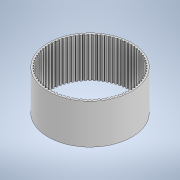
# Autodesk Inventor part: Closed Loop GT-2 (parametric)
Saved by Autodesk Inventor 2020.3 (Build 243373000, 373)
## iProperties
Created: 2021-02-16
Part Number: Closed Loop GT-2 (parametric)
Material: Generic
Document SubType Name: Modeling
Designer: juanp
Density: 1 g/cm^3
Appearance: Default
Author: juanp
Autodesk Inventor part; units mm, degrees
(part 1 of 2)
ref_plane "YZ Plane" through (0, 0, 0) normal (1, 0, 0) x (0, 1, 0)
ref_plane "XZ Plane" through (0, 0, 0) normal (0, 1, 0) x (-1, 0, 0)
ref_plane "XY Plane" through (0, 0, 0) normal (0, 0, 1) x (1, 0, 0)
sketch "Sketch1" plane through (0, 0, 0) normal (0, 1, 0) x (-1, 0, 0)
  circle A0 centre (0, 0) radius 26.3648
  circle A1 centre (0, 0) radius 25.4648
  line L0 (25.4648, 0) -> (24.7148, 0) construction
  arc A2 (25.0266, 0.4989) -> (24.7148, 0) centre (25.2698, 0) ccw
  arc A3 (25.325, 0.5902) -> (25.0266, 0.4989) centre (25.4648, -0.4) ccw
  arc A4 (25.325, 0.5902) -> (25.4539, 0.7431) centre (25.304, 0.7387) ccw
  line L1 (24.7148, 0) -> (0, 0)
  arc A5 (24.7148, 0) -> (25.0266, -0.4989) centre (25.2698, 0) ccw
  arc A6 (25.0266, -0.4989) -> (25.325, -0.5902) centre (25.4648, 0.4) ccw
  arc A7 (25.4539, -0.7431) -> (25.325, -0.5902) centre (25.304, -0.7387) ccw
  arc A8 (25.4338, 1.2563) -> (25.2932, 1.3986) centre (25.284, 1.2489) ccw
  arc A9 (24.9886, 1.4662) -> (25.2932, 1.3986) centre (25.3549, 2.3967) ccw
  arc A10 (24.6386, 1.9391) -> (24.9886, 1.4662) centre (25.1919, 1.9826) ccw
  line L2 (25.3863, 1.9979) -> (24.6386, 1.9391) construction
  arc A11 (25.2006, 2.5753) -> (24.9103, 2.4609) centre (25.4177, 1.5992) ccw
  arc A12 (24.9103, 2.4609) -> (24.6386, 1.9391) centre (25.1919, 1.9826) ccw
  arc A13 (25.2006, 2.5753) -> (25.3172, 2.7379) centre (25.168, 2.7218) ccw
  arc A14 (25.2568, 3.2479) -> (25.1055, 3.3788) centre (25.108, 3.2288) ccw
  arc A15 (24.7965, 3.4223) -> (25.1055, 3.3788) centre (25.0887, 4.3786) ccw
  arc A16 (24.4105, 3.8662) -> (24.7965, 3.4223) centre (24.9587, 3.9531) ccw
  line L3 (25.1513, 3.9836) -> (24.4105, 3.8662) construction
  arc A17 (24.9209, 4.5446) -> (24.6404, 4.4078) centre (25.2139, 3.5885) ccw
  arc A18 (24.6404, 4.4078) -> (24.4105, 3.8662) centre (24.9587, 3.9531) ccw
  arc A19 (24.9209, 4.5446) -> (25.0243, 4.7158) centre (24.8769, 4.688) ccw
  arc A20 (24.9241, 5.2196) -> (24.763, 5.3381) centre (24.7773, 5.1888) ccw
  arc A21 (24.4516, 5.3572) -> (24.763, 5.3381) centre (24.6678, 6.3336) ccw
  arc A22 (24.0319, 5.7696) -> (24.4516, 5.3572) centre (24.5716, 5.8991) ccw
  line L4 (24.7612, 5.9446) -> (24.0319, 5.7696) construction
  arc A23 (24.4875, 6.4859) -> (24.2186, 6.3274) centre (24.8546, 5.5557) ccw
  arc A24 (24.2186, 6.3274) -> (24.0319, 5.7696) centre (24.5716, 5.8991) ccw
  arc A25 (24.4875, 6.4859) -> (24.5772, 6.6647) centre (24.4324, 6.6254) ccw
  arc A26 (24.4378, 7.159) -> (24.2679, 7.2646) centre (24.2938, 7.1168) ccw
  arc A27 (23.9559, 7.2592) -> (24.2679, 7.2646) centre (24.0948, 8.2495) ccw
  arc A28 (23.5052, 7.6373) -> (23.9559, 7.2592) centre (24.033, 7.8088) ccw
  line L5 (24.2185, 7.8691) -> (23.5052, 7.6373) construction
  arc A29 (23.9031, 8.3871) -> (23.6475, 8.2081) centre (24.3421, 7.4886) ccw
  arc A30 (23.6475, 8.2081) -> (23.5052, 7.6373) centre (24.033, 7.8088) ccw
  arc A31 (23.9031, 8.3871) -> (23.9785, 8.5724) centre (23.8373, 8.5219) ccw
  arc A32 (23.8007, 9.0543) -> (23.6231, 9.1462) centre (23.6605, 9.001) ccw
  arc A33 (23.3125, 9.1164) -> (23.6231, 9.1462) centre (23.3733, 10.1145) ccw
  arc A34 (22.8335, 9.4579) -> (23.3125, 9.1164) centre (23.3462, 9.6703) ccw
  line L6 (23.5264, 9.745) -> (22.8335, 9.4579) construction
  arc A35 (23.1714, 10.2367) -> (22.9306, 10.0382) centre (23.6795, 9.3754) ccw
  arc A36 (22.9306, 10.0382) -> (22.8335, 9.4579) centre (23.3462, 9.6703) ccw
  arc A37 (23.1714, 10.2367) -> (23.232, 10.4273) centre (23.0952, 10.3659) ccw
  arc A38 (23.017, 10.8938) -> (22.8327, 10.9714) centre (22.8814, 10.8296) ccw
  arc A39 (22.5253, 10.9173) -> (22.8327, 10.9714) centre (22.5077, 11.9172) ccw
  arc A40 (22.021, 11.2203) -> (22.5253, 10.9173) centre (22.5155, 11.4722) ccw
  line L7 (22.6893, 11.5608) -> (22.021, 11.2203) construction
  arc A41 (22.2968, 12.0232) -> (22.0724, 11.8063) centre (22.8709, 11.2044) ccw
  arc A42 (22.0724, 11.8063) -> (22.021, 11.2203) centre (22.5155, 11.4722) ccw
  arc A43 (22.2968, 12.0232) -> (22.3423, 12.2179) centre (22.2107, 12.146) ccw
  arc A44 (22.0913, 12.6661) -> (21.9015, 12.7291) centre (21.9612, 12.5915) ccw
  arc A45 (21.5993, 12.651) -> (21.9015, 12.7291) centre (21.5033, 13.6464) ccw
  arc A46 (21.0728, 12.9134) -> (21.5993, 12.651) centre (21.546, 13.2034) ccw
  line L8 (21.7123, 13.3053) -> (21.0728, 12.9134) construction
  arc A47 (21.2847, 13.7355) -> (21.078, 13.5017) centre (21.9213, 12.9643) ccw
  arc A48 (21.078, 13.5017) -> (21.0728, 12.9134) centre (21.546, 13.2034) ccw
  arc A49 (21.2847, 13.7355) -> (21.3148, 13.9332) centre (21.1892, 13.8512) ccw
  arc A50 (21.0294, 14.3603) -> (20.8352, 14.4082) centre (20.9056, 14.2757) ccw
  arc A51 (20.5402, 14.3067) -> (20.8352, 14.4082) centre (20.3663, 15.2914) ccw
  arc A52 (19.9947, 14.527) -> (20.5402, 14.3067) centre (20.4437, 14.8532) ccw
  line L9 (20.6014, 14.9678) -> (19.9947, 14.527) construction
  arc A53 (20.1414, 15.3631) -> (19.9537, 15.1139) centre (20.8366, 14.6442) ccw
  arc A54 (19.9537, 15.1139) -> (19.9947, 14.527) centre (20.4437, 14.8532) ccw
  arc A55 (20.1414, 15.3631) -> (20.1559, 15.5626) centre (20.0372, 15.4709) ccw
  arc A56 (19.8379, 15.966) -> (19.6406, 15.9985) centre (19.7211, 15.8719) ccw
  arc A57 (19.3544, 15.8741) -> (19.6406, 15.9985) centre (19.1038, 16.8422) ccw
  arc A58 (18.7933, 16.051) -> (19.3544, 15.8741) centre (19.2153, 16.4114) ccw
  line L10 (19.3636, 16.5381) -> (18.7933, 16.051) construction
  arc A59 (18.874, 16.896) -> (18.7064, 16.6328) centre (19.6234, 16.2339) ccw
  arc A60 (18.7064, 16.6328) -> (18.7933, 16.051) centre (19.2153, 16.4114) ccw
  arc A61 (18.874, 16.896) -> (18.8727, 17.0961) centre (18.7616, 16.9954) ccw
  arc A62 (18.5241, 17.4732) -> (18.3248, 17.4901) centre (18.415, 17.3703) ccw
  arc A63 (18.0492, 17.3437) -> (18.3248, 17.4901) centre (17.7235, 18.2892) ccw
  arc A64 (17.476, 17.476) -> (18.0492, 17.3437) centre (17.8684, 17.8684) ccw
  line L11 (18.0063, 18.0063) -> (17.476, 17.476) construction
  arc A65 (17.4901, 18.3248) -> (17.3437, 18.0492) centre (18.2892, 17.7235) ccw
  arc A66 (17.3437, 18.0492) -> (17.476, 17.476) centre (17.8684, 17.8684) ccw
  arc A67 (17.4901, 18.3248) -> (17.4732, 18.5241) centre (17.3703, 18.415) ccw
  arc A68 (17.0961, 18.8727) -> (16.896, 18.874) centre (16.9954, 18.7616) ccw
  arc A69 (16.6328, 18.7064) -> (16.896, 18.874) centre (16.2339, 19.6234) ccw
  arc A70 (16.051, 18.7933) -> (16.6328, 18.7064) centre (16.4114, 19.2153) ccw
  line L12 (16.5381, 19.3636) -> (16.051, 18.7933) construction
  arc A71 (15.9985, 19.6406) -> (15.8741, 19.3544) centre (16.8422, 19.1038) ccw
  arc A72 (15.8741, 19.3544) -> (16.051, 18.7933) centre (16.4114, 19.2153) ccw
  arc A73 (15.9985, 19.6406) -> (15.966, 19.8379) centre (15.8719, 19.7211) ccw
  arc A74 (15.5626, 20.1559) -> (15.3631, 20.1414) centre (15.4709, 20.0372) ccw
  arc A75 (15.1139, 19.9537) -> (15.3631, 20.1414) centre (14.6442, 20.8366) ccw
  arc A76 (14.527, 19.9947) -> (15.1139, 19.9537) centre (14.8532, 20.4437) ccw
  line L13 (14.9678, 20.6014) -> (14.527, 19.9947) construction
  arc A77 (14.4082, 20.8352) -> (14.3067, 20.5402) centre (15.2914, 20.3663) ccw
  arc A78 (14.3067, 20.5402) -> (14.527, 19.9947) centre (14.8532, 20.4437) ccw
  arc A79 (14.4082, 20.8352) -> (14.3603, 21.0294) centre (14.2757, 20.9056) ccw
  arc A80 (13.9332, 21.3148) -> (13.7355, 21.2847) centre (13.8512, 21.1892) ccw
  arc A81 (13.5017, 21.078) -> (13.7355, 21.2847) centre (12.9643, 21.9213) ccw
  arc A82 (12.9134, 21.0728) -> (13.5017, 21.078) centre (13.2034, 21.546) ccw
  line L14 (13.3053, 21.7123) -> (12.9134, 21.0728) construction
  arc A83 (12.7291, 21.9015) -> (12.651, 21.5993) centre (13.6464, 21.5033) ccw
  arc A84 (12.651, 21.5993) -> (12.9134, 21.0728) centre (13.2034, 21.546) ccw
  arc A85 (12.7291, 21.9015) -> (12.6661, 22.0913) centre (12.5915, 21.9612) ccw
  arc A86 (12.2179, 22.3423) -> (12.0232, 22.2968) centre (12.146, 22.2107) ccw
  arc A87 (11.8063, 22.0724) -> (12.0232, 22.2968) centre (11.2044, 22.8709) ccw
  arc A88 (11.2203, 22.021) -> (11.8063, 22.0724) centre (11.4722, 22.5155) ccw
  line L15 (11.5608, 22.6893) -> (11.2203, 22.021) construction
  arc A89 (10.9714, 22.8327) -> (10.9173, 22.5253) centre (11.9172, 22.5077) ccw
  arc A90 (10.9173, 22.5253) -> (11.2203, 22.021) centre (11.4722, 22.5155) ccw
  arc A91 (10.9714, 22.8327) -> (10.8938, 23.017) centre (10.8296, 22.8814) ccw
  arc A92 (10.4273, 23.232) -> (10.2367, 23.1714) centre (10.3659, 23.0952) ccw
  arc A93 (10.0382, 22.9306) -> (10.2367, 23.1714) centre (9.3754, 23.6795) ccw
  arc A94 (9.4579, 22.8335) -> (10.0382, 22.9306) centre (9.6703, 23.3462) ccw
  line L16 (9.745, 23.5264) -> (9.4579, 22.8335) construction
  arc A95 (9.1462, 23.6231) -> (9.1164, 23.3125) centre (10.1145, 23.3733) ccw
  arc A96 (9.1164, 23.3125) -> (9.4579, 22.8335) centre (9.6703, 23.3462) ccw
  arc A97 (9.1462, 23.6231) -> (9.0543, 23.8007) centre (9.001, 23.6605) ccw
  arc A98 (8.5724, 23.9785) -> (8.3871, 23.9031) centre (8.5219, 23.8373) ccw
  arc A99 (8.2081, 23.6475) -> (8.3871, 23.9031) centre (7.4886, 24.3421) ccw
  arc A100 (7.6373, 23.5052) -> (8.2081, 23.6475) centre (7.8088, 24.033) ccw
  line L17 (7.8691, 24.2185) -> (7.6373, 23.5052) construction
  arc A101 (7.2646, 24.2679) -> (7.2592, 23.9559) centre (8.2495, 24.0948) ccw
  arc A102 (7.2592, 23.9559) -> (7.6373, 23.5052) centre (7.8088, 24.033) ccw
  arc A103 (7.2646, 24.2679) -> (7.159, 24.4378) centre (7.1168, 24.2938) ccw
  arc A104 (6.6647, 24.5772) -> (6.4859, 24.4875) centre (6.6254, 24.4324) ccw
  arc A105 (6.3274, 24.2186) -> (6.4859, 24.4875) centre (5.5557, 24.8546) ccw
  arc A106 (5.7696, 24.0319) -> (6.3274, 24.2186) centre (5.8991, 24.5716) ccw
  line L18 (5.9446, 24.7612) -> (5.7696, 24.0319) construction
  arc A107 (5.3381, 24.763) -> (5.3572, 24.4516) centre (6.3336, 24.6678) ccw
  arc A108 (5.3572, 24.4516) -> (5.7696, 24.0319) centre (5.8991, 24.5716) ccw
  arc A109 (5.3381, 24.763) -> (5.2196, 24.9241) centre (5.1888, 24.7773) ccw
  arc A110 (4.7158, 25.0243) -> (4.5446, 24.9209) centre (4.688, 24.8769) ccw
  arc A111 (4.4078, 24.6404) -> (4.5446, 24.9209) centre (3.5885, 25.2139) ccw
  arc A112 (3.8662, 24.4105) -> (4.4078, 24.6404) centre (3.9531, 24.9587) ccw
  line L19 (3.9836, 25.1513) -> (3.8662, 24.4105) construction
  arc A113 (3.3788, 25.1055) -> (3.4223, 24.7965) centre (4.3786, 25.0887) ccw
  arc A114 (3.4223, 24.7965) -> (3.8662, 24.4105) centre (3.9531, 24.9587) ccw
  arc A115 (3.3788, 25.1055) -> (3.2479, 25.2568) centre (3.2288, 25.108) ccw
  arc A116 (2.7379, 25.3172) -> (2.5753, 25.2006) centre (2.7218, 25.168) ccw
  arc A117 (2.4609, 24.9103) -> (2.5753, 25.2006) centre (1.5992, 25.4177) ccw
  arc A118 (1.9391, 24.6386) -> (2.4609, 24.9103) centre (1.9826, 25.1919) ccw
  line L20 (1.9979, 25.3863) -> (1.9391, 24.6386) construction
  arc A119 (1.3986, 25.2932) -> (1.4662, 24.9886) centre (2.3967, 25.3549) ccw
  arc A120 (1.4662, 24.9886) -> (1.9391, 24.6386) centre (1.9826, 25.1919) ccw
  arc A121 (1.3986, 25.2932) -> (1.2563, 25.4338) centre (1.2489, 25.284) ccw
  arc A122 (0.7431, 25.4539) -> (0.5902, 25.325) centre (0.7387, 25.304) ccw
  arc A123 (0.4989, 25.0266) -> (0.5902, 25.325) centre (-0.4, 25.4648) ccw
  arc A124 (0, 24.7148) -> (0.4989, 25.0266) centre (0, 25.2698) ccw
  line L21 (0, 25.4648) -> (0, 24.7148) construction
  arc A125 (-0.5902, 25.325) -> (-0.4989, 25.0266) centre (0.4, 25.4648) ccw
  arc A126 (-0.4989, 25.0266) -> (0, 24.7148) centre (0, 25.2698) ccw
  arc A127 (-0.5902, 25.325) -> (-0.7431, 25.4539) centre (-0.7387, 25.304) ccw
  arc A128 (-1.2563, 25.4338) -> (-1.3986, 25.2932) centre (-1.2489, 25.284) ccw
  arc A129 (-1.4662, 24.9886) -> (-1.3986, 25.2932) centre (-2.3967, 25.3549) ccw
  arc A130 (-1.9391, 24.6386) -> (-1.4662, 24.9886) centre (-1.9826, 25.1919) ccw
  line L22 (-1.9979, 25.3863) -> (-1.9391, 24.6386) construction
  arc A131 (-2.5753, 25.2006) -> (-2.4609, 24.9103) centre (-1.5992, 25.4177) ccw
  arc A132 (-2.4609, 24.9103) -> (-1.9391, 24.6386) centre (-1.9826, 25.1919) ccw
  arc A133 (-2.5753, 25.2006) -> (-2.7379, 25.3172) centre (-2.7218, 25.168) ccw
  arc A134 (-3.2479, 25.2568) -> (-3.3788, 25.1055) centre (-3.2288, 25.108) ccw
  arc A135 (-3.4223, 24.7965) -> (-3.3788, 25.1055) centre (-4.3786, 25.0887) ccw
  arc A136 (-3.8662, 24.4105) -> (-3.4223, 24.7965) centre (-3.9531, 24.9587) ccw
  line L23 (-3.9836, 25.1513) -> (-3.8662, 24.4105) construction
  arc A137 (-4.5446, 24.9209) -> (-4.4078, 24.6404) centre (-3.5885, 25.2139) ccw
  arc A138 (-4.4078, 24.6404) -> (-3.8662, 24.4105) centre (-3.9531, 24.9587) ccw
  arc A139 (-4.5446, 24.9209) -> (-4.7158, 25.0243) centre (-4.688, 24.8769) ccw
  arc A140 (-5.2196, 24.9241) -> (-5.3381, 24.763) centre (-5.1888, 24.7773) ccw
  arc A141 (-5.3572, 24.4516) -> (-5.3381, 24.763) centre (-6.3336, 24.6678) ccw
  arc A142 (-5.7696, 24.0319) -> (-5.3572, 24.4516) centre (-5.8991, 24.5716) ccw
  line L24 (-5.9446, 24.7612) -> (-5.7696, 24.0319) construction
  arc A143 (-6.4859, 24.4875) -> (-6.3274, 24.2186) centre (-5.5557, 24.8546) ccw
  arc A144 (-6.3274, 24.2186) -> (-5.7696, 24.0319) centre (-5.8991, 24.5716) ccw
  arc A145 (-6.4859, 24.4875) -> (-6.6647, 24.5772) centre (-6.6254, 24.4324) ccw
  arc A146 (-7.159, 24.4378) -> (-7.2646, 24.2679) centre (-7.1168, 24.2938) ccw
  arc A147 (-7.2592, 23.9559) -> (-7.2646, 24.2679) centre (-8.2495, 24.0948) ccw
  arc A148 (-7.6373, 23.5052) -> (-7.2592, 23.9559) centre (-7.8088, 24.033) ccw
  line L25 (-7.8691, 24.2185) -> (-7.6373, 23.5052) construction
  arc A149 (-8.3871, 23.9031) -> (-8.2081, 23.6475) centre (-7.4886, 24.3421) ccw
  arc A150 (-8.2081, 23.6475) -> (-7.6373, 23.5052) centre (-7.8088, 24.033) ccw
  arc A151 (-8.3871, 23.9031) -> (-8.5724, 23.9785) centre (-8.5219, 23.8373) ccw
  arc A152 (-9.0543, 23.8007) -> (-9.1462, 23.6231) centre (-9.001, 23.6605) ccw
  arc A153 (-9.1164, 23.3125) -> (-9.1462, 23.6231) centre (-10.1145, 23.3733) ccw
  arc A154 (-9.4579, 22.8335) -> (-9.1164, 23.3125) centre (-9.6703, 23.3462) ccw
  line L26 (-9.745, 23.5264) -> (-9.4579, 22.8335) construction
  arc A155 (-10.2367, 23.1714) -> (-10.0382, 22.9306) centre (-9.3754, 23.6795) ccw
  arc A156 (-10.0382, 22.9306) -> (-9.4579, 22.8335) centre (-9.6703, 23.3462) ccw
  arc A157 (-10.2367, 23.1714) -> (-10.4273, 23.232) centre (-10.3659, 23.0952) ccw
  arc A158 (-10.8938, 23.017) -> (-10.9714, 22.8327) centre (-10.8296, 22.8814) ccw
  arc A159 (-10.9173, 22.5253) -> (-10.9714, 22.8327) centre (-11.9172, 22.5077) ccw
  arc A160 (-11.2203, 22.021) -> (-10.9173, 22.5253) centre (-11.4722, 22.5155) ccw
  line L27 (-11.5608, 22.6893) -> (-11.2203, 22.021) construction
  arc A161 (-12.0232, 22.2968) -> (-11.8063, 22.0724) centre (-11.2044, 22.8709) ccw
  arc A162 (-11.8063, 22.0724) -> (-11.2203, 22.021) centre (-11.4722, 22.5155) ccw
  arc A163 (-12.0232, 22.2968) -> (-12.2179, 22.3423) centre (-12.146, 22.2107) ccw
  arc A164 (-12.6661, 22.0913) -> (-12.7291, 21.9015) centre (-12.5915, 21.9612) ccw
  arc A165 (-12.651, 21.5993) -> (-12.7291, 21.9015) centre (-13.6464, 21.5033) ccw
  arc A166 (-12.9134, 21.0728) -> (-12.651, 21.5993) centre (-13.2034, 21.546) ccw
  line L28 (-13.3053, 21.7123) -> (-12.9134, 21.0728) construction
  arc A167 (-13.7355, 21.2847) -> (-13.5017, 21.078) centre (-12.9643, 21.9213) ccw
  arc A168 (-13.5017, 21.078) -> (-12.9134, 21.0728) centre (-13.2034, 21.546) ccw
  arc A169 (-13.7355, 21.2847) -> (-13.9332, 21.3148) centre (-13.8512, 21.1892) ccw
  arc A170 (-14.3603, 21.0294) -> (-14.4082, 20.8352) centre (-14.2757, 20.9056) ccw
  arc A171 (-14.3067, 20.5402) -> (-14.4082, 20.8352) centre (-15.2914, 20.3663) ccw
  arc A172 (-14.527, 19.9947) -> (-14.3067, 20.5402) centre (-14.8532, 20.4437) ccw
  line L29 (-14.9678, 20.6014) -> (-14.527, 19.9947) construction
  arc A173 (-15.3631, 20.1414) -> (-15.1139, 19.9537) centre (-14.6442, 20.8366) ccw
  arc A174 (-15.1139, 19.9537) -> (-14.527, 19.9947) centre (-14.8532, 20.4437) ccw
  arc A175 (-15.3631, 20.1414) -> (-15.5626, 20.1559) centre (-15.4709, 20.0372) ccw
  arc A176 (-15.966, 19.8379) -> (-15.9985, 19.6406) centre (-15.8719, 19.7211) ccw
  arc A177 (-15.8741, 19.3544) -> (-15.9985, 19.6406) centre (-16.8422, 19.1038) ccw
  arc A178 (-16.051, 18.7933) -> (-15.8741, 19.3544) centre (-16.4114, 19.2153) ccw
  line L30 (-16.5381, 19.3636) -> (-16.051, 18.7933) construction
  arc A179 (-16.896, 18.874) -> (-16.6328, 18.7064) centre (-16.2339, 19.6234) ccw
  arc A180 (-16.6328, 18.7064) -> (-16.051, 18.7933) centre (-16.4114, 19.2153) ccw
  arc A181 (-16.896, 18.874) -> (-17.0961, 18.8727) centre (-16.9954, 18.7616) ccw
  arc A182 (-17.4732, 18.5241) -> (-17.4901, 18.3248) centre (-17.3703, 18.415) ccw
  arc A183 (-17.3437, 18.0492) -> (-17.4901, 18.3248) centre (-18.2892, 17.7235) ccw
  arc A184 (-17.476, 17.476) -> (-17.3437, 18.0492) centre (-17.8684, 17.8684) ccw
  line L31 (-18.0063, 18.0063) -> (-17.476, 17.476) construction
  arc A185 (-18.3248, 17.4901) -> (-18.0492, 17.3437) centre (-17.7235, 18.2892) ccw
  arc A186 (-18.0492, 17.3437) -> (-17.476, 17.476) centre (-17.8684, 17.8684) ccw
  arc A187 (-18.3248, 17.4901) -> (-18.5241, 17.4732) centre (-18.415, 17.3703) ccw
  arc A188 (-18.8727, 17.0961) -> (-18.874, 16.896) centre (-18.7616, 16.9954) ccw
  arc A189 (-18.7064, 16.6328) -> (-18.874, 16.896) centre (-19.6234, 16.2339) ccw
  arc A190 (-18.7933, 16.051) -> (-18.7064, 16.6328) centre (-19.2153, 16.4114) ccw
  line L32 (-19.3636, 16.5381) -> (-18.7933, 16.051) construction
  arc A191 (-19.6406, 15.9985) -> (-19.3544, 15.8741) centre (-19.1038, 16.8422) ccw
  arc A192 (-19.3544, 15.8741) -> (-18.7933, 16.051) centre (-19.2153, 16.4114) ccw
  arc A193 (-19.6406, 15.9985) -> (-19.8379, 15.966) centre (-19.7211, 15.8719) ccw
  arc A194 (-20.1559, 15.5626) -> (-20.1414, 15.3631) centre (-20.0372, 15.4709) ccw
  arc A195 (-19.9537, 15.1139) -> (-20.1414, 15.3631) centre (-20.8366, 14.6442) ccw
  arc A196 (-19.9947, 14.527) -> (-19.9537, 15.1139) centre (-20.4437, 14.8532) ccw
  line L33 (-20.6014, 14.9678) -> (-19.9947, 14.527) construction
  arc A197 (-20.8352, 14.4082) -> (-20.5402, 14.3067) centre (-20.3663, 15.2914) ccw
  arc A198 (-20.5402, 14.3067) -> (-19.9947, 14.527) centre (-20.4437, 14.8532) ccw
  arc A199 (-20.8352, 14.4082) -> (-21.0294, 14.3603) centre (-20.9056, 14.2757) ccw
  arc A200 (-21.3148, 13.9332) -> (-21.2847, 13.7355) centre (-21.1892, 13.8512) ccw
  arc A201 (-21.078, 13.5017) -> (-21.2847, 13.7355) centre (-21.9213, 12.9643) ccw
  arc A202 (-21.0728, 12.9134) -> (-21.078, 13.5017) centre (-21.546, 13.2034) ccw
  line L34 (-21.7123, 13.3053) -> (-21.0728, 12.9134) construction
  arc A203 (-21.9015, 12.7291) -> (-21.5993, 12.651) centre (-21.5033, 13.6464) ccw
  arc A204 (-21.5993, 12.651) -> (-21.0728, 12.9134) centre (-21.546, 13.2034) ccw
  arc A205 (-21.9015, 12.7291) -> (-22.0913, 12.6661) centre (-21.9612, 12.5915) ccw
  arc A206 (-22.3423, 12.2179) -> (-22.2968, 12.0232) centre (-22.2107, 12.146) ccw
  arc A207 (-22.0724, 11.8063) -> (-22.2968, 12.0232) centre (-22.8709, 11.2044) ccw
  arc A208 (-22.021, 11.2203) -> (-22.0724, 11.8063) centre (-22.5155, 11.4722) ccw
  line L35 (-22.6893, 11.5608) -> (-22.021, 11.2203) construction
  arc A209 (-22.8327, 10.9714) -> (-22.5253, 10.9173) centre (-22.5077, 11.9172) ccw
  arc A210 (-22.5253, 10.9173) -> (-22.021, 11.2203) centre (-22.5155, 11.4722) ccw
  arc A211 (-22.8327, 10.9714) -> (-23.017, 10.8938) centre (-22.8814, 10.8296) ccw
  arc A212 (-23.232, 10.4273) -> (-23.1714, 10.2367) centre (-23.0952, 10.3659) ccw
  arc A213 (-22.9306, 10.0382) -> (-23.1714, 10.2367) centre (-23.6795, 9.3754) ccw
  arc A214 (-22.8335, 9.4579) -> (-22.9306, 10.0382) centre (-23.3462, 9.6703) ccw
  line L36 (-23.5264, 9.745) -> (-22.8335, 9.4579) construction
  arc A215 (-23.6231, 9.1462) -> (-23.3125, 9.1164) centre (-23.3733, 10.1145) ccw
  arc A216 (-23.3125, 9.1164) -> (-22.8335, 9.4579) centre (-23.3462, 9.6703) ccw
  arc A217 (-23.6231, 9.1462) -> (-23.8007, 9.0543) centre (-23.6605, 9.001) ccw
  arc A218 (-23.9785, 8.5724) -> (-23.9031, 8.3871) centre (-23.8373, 8.5219) ccw
  arc A219 (-23.6475, 8.2081) -> (-23.9031, 8.3871) centre (-24.3421, 7.4886) ccw
  arc A220 (-23.5052, 7.6373) -> (-23.6475, 8.2081) centre (-24.033, 7.8088) ccw
  line L37 (-24.2185, 7.8691) -> (-23.5052, 7.6373) construction
  arc A221 (-24.2679, 7.2646) -> (-23.9559, 7.2592) centre (-24.0948, 8.2495) ccw
  arc A222 (-23.9559, 7.2592) -> (-23.5052, 7.6373) centre (-24.033, 7.8088) ccw
  arc A223 (-24.2679, 7.2646) -> (-24.4378, 7.159) centre (-24.2938, 7.1168) ccw
  arc A224 (-24.5772, 6.6647) -> (-24.4875, 6.4859) centre (-24.4324, 6.6254) ccw
  arc A225 (-24.2186, 6.3274) -> (-24.4875, 6.4859) centre (-24.8546, 5.5557) ccw
  arc A226 (-24.0319, 5.7696) -> (-24.2186, 6.3274) centre (-24.5716, 5.8991) ccw
  line L38 (-24.7612, 5.9446) -> (-24.0319, 5.7696) construction
  arc A227 (-24.763, 5.3381) -> (-24.4516, 5.3572) centre (-24.6678, 6.3336) ccw
  arc A228 (-24.4516, 5.3572) -> (-24.0319, 5.7696) centre (-24.5716, 5.8991) ccw
  arc A229 (-24.763, 5.3381) -> (-24.9241, 5.2196) centre (-24.7773, 5.1888) ccw
  arc A230 (-25.0243, 4.7158) -> (-24.9209, 4.5446) centre (-24.8769, 4.688) ccw
  arc A231 (-24.6404, 4.4078) -> (-24.9209, 4.5446) centre (-25.2139, 3.5885) ccw
  arc A232 (-24.4105, 3.8662) -> (-24.6404, 4.4078) centre (-24.9587, 3.9531) ccw
  line L39 (-25.1513, 3.9836) -> (-24.4105, 3.8662) construction
  arc A233 (-25.1055, 3.3788) -> (-24.7965, 3.4223) centre (-25.0887, 4.3786) ccw
  arc A234 (-24.7965, 3.4223) -> (-24.4105, 3.8662) centre (-24.9587, 3.9531) ccw
  arc A235 (-25.1055, 3.3788) -> (-25.2568, 3.2479) centre (-25.108, 3.2288) ccw
  arc A236 (-25.3172, 2.7379) -> (-25.2006, 2.5753) centre (-25.168, 2.7218) ccw
  arc A237 (-24.9103, 2.4609) -> (-25.2006, 2.5753) centre (-25.4177, 1.5992) ccw
  arc A238 (-24.6386, 1.9391) -> (-24.9103, 2.4609) centre (-25.1919, 1.9826) ccw
  line L40 (-25.3863, 1.9979) -> (-24.6386, 1.9391) construction
  arc A239 (-25.2932, 1.3986) -> (-24.9886, 1.4662) centre (-25.3549, 2.3967) ccw
  arc A240 (-24.9886, 1.4662) -> (-24.6386, 1.9391) centre (-25.1919, 1.9826) ccw
  arc A241 (-25.2932, 1.3986) -> (-25.4338, 1.2563) centre (-25.284, 1.2489) ccw
  arc A242 (-25.4539, 0.7431) -> (-25.325, 0.5902) centre (-25.304, 0.7387) ccw
  arc A243 (-25.0266, 0.4989) -> (-25.325, 0.5902) centre (-25.4648, -0.4) ccw
  arc A244 (-24.7148, 0) -> (-25.0266, 0.4989) centre (-25.2698, 0) ccw
  line L41 (-25.4648, 0) -> (-24.7148, 0) construction
  arc A245 (-25.325, -0.5902) -> (-25.0266, -0.4989) centre (-25.4648, 0.4) ccw
  arc A246 (-25.0266, -0.4989) -> (-24.7148, 0) centre (-25.2698, 0) ccw
  arc A247 (-25.325, -0.5902) -> (-25.4539, -0.7431) centre (-25.304, -0.7387) ccw
  arc A248 (-25.4338, -1.2563) -> (-25.2932, -1.3986) centre (-25.284, -1.2489) ccw
  arc A249 (-24.9886, -1.4662) -> (-25.2932, -1.3986) centre (-25.3549, -2.3967) ccw
  arc A250 (-24.6386, -1.9391) -> (-24.9886, -1.4662) centre (-25.1919, -1.9826) ccw
  line L42 (-25.3863, -1.9979) -> (-24.6386, -1.9391) construction
  arc A251 (-25.2006, -2.5753) -> (-24.9103, -2.4609) centre (-25.4177, -1.5992) ccw
  arc A252 (-24.9103, -2.4609) -> (-24.6386, -1.9391) centre (-25.1919, -1.9826) ccw
  arc A253 (-25.2006, -2.5753) -> (-25.3172, -2.7379) centre (-25.168, -2.7218) ccw
  arc A254 (-25.2568, -3.2479) -> (-25.1055, -3.3788) centre (-25.108, -3.2288) ccw
  arc A255 (-24.7965, -3.4223) -> (-25.1055, -3.3788) centre (-25.0887, -4.3786) ccw
  arc A256 (-24.4105, -3.8662) -> (-24.7965, -3.4223) centre (-24.9587, -3.9531) ccw
  line L43 (-25.1513, -3.9836) -> (-24.4105, -3.8662) construction
  arc A257 (-24.9209, -4.5446) -> (-24.6404, -4.4078) centre (-25.2139, -3.5885) ccw
  arc A258 (-24.6404, -4.4078) -> (-24.4105, -3.8662) centre (-24.9587, -3.9531) ccw
  arc A259 (-24.9209, -4.5446) -> (-25.0243, -4.7158) centre (-24.8769, -4.688) ccw
  arc A260 (-24.9241, -5.2196) -> (-24.763, -5.3381) centre (-24.7773, -5.1888) ccw
  arc A261 (-24.4516, -5.3572) -> (-24.763, -5.3381) centre (-24.6678, -6.3336) ccw
  arc A262 (-24.0319, -5.7696) -> (-24.4516, -5.3572) centre (-24.5716, -5.8991) ccw
  line L44 (-24.7612, -5.9446) -> (-24.0319, -5.7696) construction
  arc A263 (-24.4875, -6.4859) -> (-24.2186, -6.3274) centre (-24.8546, -5.5557) ccw
  arc A264 (-24.2186, -6.3274) -> (-24.0319, -5.7696) centre (-24.5716, -5.8991) ccw
  arc A265 (-24.4875, -6.4859) -> (-24.5772, -6.6647) centre (-24.4324, -6.6254) ccw
  arc A266 (-24.4378, -7.159) -> (-24.2679, -7.2646) centre (-24.2938, -7.1168) ccw
  arc A267 (-23.9559, -7.2592) -> (-24.2679, -7.2646) centre (-24.0948, -8.2495) ccw
  arc A268 (-23.5052, -7.6373) -> (-23.9559, -7.2592) centre (-24.033, -7.8088) ccw
  line L45 (-24.2185, -7.8691) -> (-23.5052, -7.6373) construction
  arc A269 (-23.9031, -8.3871) -> (-23.6475, -8.2081) centre (-24.3421, -7.4886) ccw
  arc A270 (-23.6475, -8.2081) -> (-23.5052, -7.6373) centre (-24.033, -7.8088) ccw
  arc A271 (-23.9031, -8.3871) -> (-23.9785, -8.5724) centre (-23.8373, -8.5219) ccw
  arc A272 (-23.8007, -9.0543) -> (-23.6231, -9.1462) centre (-23.6605, -9.001) ccw
  arc A273 (-23.3125, -9.1164) -> (-23.6231, -9.1462) centre (-23.3733, -10.1145) ccw
  arc A274 (-22.8335, -9.4579) -> (-23.3125, -9.1164) centre (-23.3462, -9.6703) ccw
  line L46 (-23.5264, -9.745) -> (-22.8335, -9.4579) construction
  arc A275 (-23.1714, -10.2367) -> (-22.9306, -10.0382) centre (-23.6795, -9.3754) ccw
  arc A276 (-22.9306, -10.0382) -> (-22.8335, -9.4579) centre (-23.3462, -9.6703) ccw
  arc A277 (-23.1714, -10.2367) -> (-23.232, -10.4273) centre (-23.0952, -10.3659) ccw
  arc A278 (-23.017, -10.8938) -> (-22.8327, -10.9714) centre (-22.8814, -10.8296) ccw
  arc A279 (-22.5253, -10.9173) -> (-22.8327, -10.9714) centre (-22.5077, -11.9172) ccw
  arc A280 (-22.021, -11.2203) -> (-22.5253, -10.9173) centre (-22.5155, -11.4722) ccw
  line L47 (-22.6893, -11.5608) -> (-22.021, -11.2203) construction
  arc A281 (-22.2968, -12.0232) -> (-22.0724, -11.8063) centre (-22.8709, -11.2044) ccw
  arc A282 (-22.0724, -11.8063) -> (-22.021, -11.2203) centre (-22.5155, -11.4722) ccw
  arc A283 (-22.2968, -12.0232) -> (-22.3423, -12.2179) centre (-22.2107, -12.146) ccw
  arc A284 (-22.0913, -12.6661) -> (-21.9015, -12.7291) centre (-21.9612, -12.5915) ccw
  arc A285 (-21.5993, -12.651) -> (-21.9015, -12.7291) centre (-21.5033, -13.6464) ccw
  arc A286 (-21.0728, -12.9134) -> (-21.5993, -12.651) centre (-21.546, -13.2034) ccw
  line L48 (-21.7123, -13.3053) -> (-21.0728, -12.9134) construction
  arc A287 (-21.2847, -13.7355) -> (-21.078, -13.5017) centre (-21.9213, -12.9643) ccw
  arc A288 (-21.078, -13.5017) -> (-21.0728, -12.9134) centre (-21.546, -13.2034) ccw
  arc A289 (-21.2847, -13.7355) -> (-21.3148, -13.9332) centre (-21.1892, -13.8512) ccw
  arc A290 (-21.0294, -14.3603) -> (-20.8352, -14.4082) centre (-20.9056, -14.2757) ccw
  arc A291 (-20.5402, -14.3067) -> (-20.8352, -14.4082) centre (-20.3663, -15.2914) ccw
  arc A292 (-19.9947, -14.527) -> (-20.5402, -14.3067) centre (-20.4437, -14.8532) ccw
  line L49 (-20.6014, -14.9678) -> (-19.9947, -14.527) construction
  arc A293 (-20.1414, -15.3631) -> (-19.9537, -15.1139) centre (-20.8366, -14.6442) ccw
  arc A294 (-19.9537, -15.1139) -> (-19.9947, -14.527) centre (-20.4437, -14.8532) ccw
  arc A295 (-20.1414, -15.3631) -> (-20.1559, -15.5626) centre (-20.0372, -15.4709) ccw
  arc A296 (-19.8379, -15.966) -> (-19.6406, -15.9985) centre (-19.7211, -15.8719) ccw
  arc A297 (-19.3544, -15.8741) -> (-19.6406, -15.9985) centre (-19.1038, -16.8422) ccw
  arc A298 (-18.7933, -16.051) -> (-19.3544, -15.8741) centre (-19.2153, -16.4114) ccw
  line L50 (-19.3636, -16.5381) -> (-18.7933, -16.051) construction
  arc A299 (-18.874, -16.896) -> (-18.7064, -16.6328) centre (-19.6234, -16.2339) ccw
  arc A300 (-18.7064, -16.6328) -> (-18.7933, -16.051) centre (-19.2153, -16.4114) ccw
  arc A301 (-18.874, -16.896) -> (-18.8727, -17.0961) centre (-18.7616, -16.9954) ccw
  arc A302 (-18.5241, -17.4732) -> (-18.3248, -17.4901) centre (-18.415, -17.3703) ccw
  arc A303 (-18.0492, -17.3437) -> (-18.3248, -17.4901) centre (-17.7235, -18.2892) ccw
  arc A304 (-17.476, -17.476) -> (-18.0492, -17.3437) centre (-17.8684, -17.8684) ccw
  line L51 (-18.0063, -18.0063) -> (-17.476, -17.476) construction
  arc A305 (-17.4901, -18.3248) -> (-17.3437, -18.0492) centre (-18.2892, -17.7235) ccw
  arc A306 (-17.3437, -18.0492) -> (-17.476, -17.476) centre (-17.8684, -17.8684) ccw
  arc A307 (-17.4901, -18.3248) -> (-17.4732, -18.5241) centre (-17.3703, -18.415) ccw
  arc A308 (-17.0961, -18.8727) -> (-16.896, -18.874) centre (-16.9954, -18.7616) ccw
  arc A309 (-16.6328, -18.7064) -> (-16.896, -18.874) centre (-16.2339, -19.6234) ccw
  arc A310 (-16.051, -18.7933) -> (-16.6328, -18.7064) centre (-16.4114, -19.2153) ccw
  line L52 (-16.5381, -19.3636) -> (-16.051, -18.7933) construction
  arc A311 (-15.9985, -19.6406) -> (-15.8741, -19.3544) centre (-16.8422, -19.1038) ccw
  arc A312 (-15.8741, -19.3544) -> (-16.051, -18.7933) centre (-16.4114, -19.2153) ccw
  arc A313 (-15.9985, -19.6406) -> (-15.966, -19.8379) centre (-15.8719, -19.7211) ccw
  arc A314 (-15.5626, -20.1559) -> (-15.3631, -20.1414) centre (-15.4709, -20.0372) ccw
  arc A315 (-15.1139, -19.9537) -> (-15.3631, -20.1414) centre (-14.6442, -20.8366) ccw
  arc A316 (-14.527, -19.9947) -> (-15.1139, -19.9537) centre (-14.8532, -20.4437) ccw
  line L53 (-14.9678, -20.6014) -> (-14.527, -19.9947) construction
  arc A317 (-14.4082, -20.8352) -> (-14.3067, -20.5402) centre (-15.2914, -20.3663) ccw
  arc A318 (-14.3067, -20.5402) -> (-14.527, -19.9947) centre (-14.8532, -20.4437) ccw
  arc A319 (-14.4082, -20.8352) -> (-14.3603, -21.0294) centre (-14.2757, -20.9056) ccw
  arc A320 (-13.9332, -21.3148) -> (-13.7355, -21.2847) centre (-13.8512, -21.1892) ccw
  arc A321 (-13.5017, -21.078) -> (-13.7355, -21.2847) centre (-12.9643, -21.9213) ccw
  arc A322 (-12.9134, -21.0728) -> (-13.5017, -21.078) centre (-13.2034, -21.546) ccw
  line L54 (-13.3053, -21.7123) -> (-12.9134, -21.0728) construction
  arc A323 (-12.7291, -21.9015) -> (-12.651, -21.5993) centre (-13.6464, -21.5033) ccw
  arc A324 (-12.651, -21.5993) -> (-12.9134, -21.0728) centre (-13.2034, -21.546) ccw
  arc A325 (-12.7291, -21.9015) -> (-12.6661, -22.0913) centre (-12.5915, -21.9612) ccw
  arc A326 (-12.2179, -22.3423) -> (-12.0232, -22.2968) centre (-12.146, -22.2107) ccw
  arc A327 (-11.8063, -22.0724) -> (-12.0232, -22.2968) centre (-11.2044, -22.8709) ccw
  arc A328 (-11.2203, -22.021) -> (-11.8063, -22.0724) centre (-11.4722, -22.5155) ccw
  line L55 (-11.5608, -22.6893) -> (-11.2203, -22.021) construction
  arc A329 (-10.9714, -22.8327) -> (-10.9173, -22.5253) centre (-11.9172, -22.5077) ccw
  arc A330 (-10.9173, -22.5253) -> (-11.2203, -22.021) centre (-11.4722, -22.5155) ccw
  arc A331 (-10.9714, -22.8327) -> (-10.8938, -23.017) centre (-10.8296, -22.8814) ccw
  arc A332 (-10.4273, -23.232) -> (-10.2367, -23.1714) centre (-10.3659, -23.0952) ccw
  arc A333 (-10.0382, -22.9306) -> (-10.2367, -23.1714) centre (-9.3754, -23.6795) ccw
  arc A334 (-9.4579, -22.8335) -> (-10.0382, -22.9306) centre (-9.6703, -23.3462) ccw
  line L56 (-9.745, -23.5264) -> (-9.4579, -22.8335) construction
  arc A335 (-9.1462, -23.6231) -> (-9.1164, -23.3125) centre (-10.1145, -23.3733) ccw
  arc A336 (-9.1164, -23.3125) -> (-9.4579, -22.8335) centre (-9.6703, -23.3462) ccw
  arc A337 (-9.1462, -23.6231) -> (-9.0543, -23.8007) centre (-9.001, -23.6605) ccw
  arc A338 (-8.5724, -23.9785) -> (-8.3871, -23.9031) centre (-8.5219, -23.8373) ccw
  arc A339 (-8.2081, -23.6475) -> (-8.3871, -23.9031) centre (-7.4886, -24.3421) ccw
  arc A340 (-7.6373, -23.5052) -> (-8.2081, -23.6475) centre (-7.8088, -24.033) ccw
  line L57 (-7.8691, -24.2185) -> (-7.6373, -23.5052) construction
  arc A341 (-7.2646, -24.2679) -> (-7.2592, -23.9559) centre (-8.2495, -24.0948) ccw
  arc A342 (-7.2592, -23.9559) -> (-7.6373, -23.5052) centre (-7.8088, -24.033) ccw
  arc A343 (-7.2646, -24.2679) -> (-7.159, -24.4378) centre (-7.1168, -24.2938) ccw
  arc A344 (-6.6647, -24.5772) -> (-6.4859, -24.4875) centre (-6.6254, -24.4324) ccw
  arc A345 (-6.3274, -24.2186) -> (-6.4859, -24.4875) centre (-5.5557, -24.8546) ccw
  arc A346 (-5.7696, -24.0319) -> (-6.3274, -24.2186) centre (-5.8991, -24.5716) ccw
  line L58 (-5.9446, -24.7612) -> (-5.7696, -24.0319) construction
  arc A347 (-5.3381, -24.763) -> (-5.3572, -24.4516) centre (-6.3336, -24.6678) ccw
  arc A348 (-5.3572, -24.4516) -> (-5.7696, -24.0319) centre (-5.8991, -24.5716) ccw
  arc A349 (-5.3381, -24.763) -> (-5.2196, -24.9241) centre (-5.1888, -24.7773) ccw
  arc A350 (-4.7158, -25.0243) -> (-4.5446, -24.9209) centre (-4.688, -24.8769) ccw
  arc A351 (-4.4078, -24.6404) -> (-4.5446, -24.9209) centre (-3.5885, -25.2139) ccw
  arc A352 (-3.8662, -24.4105) -> (-4.4078, -24.6404) centre (-3.9531, -24.9587) ccw
  line L59 (-3.9836, -25.1513) -> (-3.8662, -24.4105) construction
  arc A353 (-3.3788, -25.1055) -> (-3.4223, -24.7965) centre (-4.3786, -25.0887) ccw
  arc A354 (-3.4223, -24.7965) -> (-3.8662, -24.4105) centre (-3.9531, -24.9587) ccw
  arc A355 (-3.3788, -25.1055) -> (-3.2479, -25.2568) centre (-3.2288, -25.108) ccw
  arc A356 (-2.7379, -25.3172) -> (-2.5753, -25.2006) centre (-2.7218, -25.168) ccw
  arc A357 (-2.4609, -24.9103) -> (-2.5753, -25.2006) centre (-1.5992, -25.4177) ccw
  arc A358 (-1.9391, -24.6386) -> (-2.4609, -24.9103) centre (-1.9826, -25.1919) ccw
  line L60 (-1.9979, -25.3863) -> (-1.9391, -24.6386) construction
  arc A359 (-1.3986, -25.2932) -> (-1.4662, -24.9886) centre (-2.3967, -25.3549) ccw
  arc A360 (-1.4662, -24.9886) -> (-1.9391, -24.6386) centre (-1.9826, -25.1919) ccw
  arc A361 (-1.3986, -25.2932) -> (-1.2563, -25.4338) centre (-1.2489, -25.284) ccw
  arc A362 (-0.7431, -25.4539) -> (-0.5902, -25.325) centre (-0.7387, -25.304) ccw
  arc A363 (-0.4989, -25.0266) -> (-0.5902, -25.325) centre (0.4, -25.4648) ccw
  arc A364 (0, -24.7148) -> (-0.4989, -25.0266) centre (0, -25.2698) ccw
  line L61 (0, -25.4648) -> (0, -24.7148) construction
  arc A365 (0.5902, -25.325) -> (0.4989, -25.0266) centre (-0.4, -25.4648) ccw
  arc A366 (0.4989, -25.0266) -> (0, -24.7148) centre (0, -25.2698) ccw
  arc A367 (0.5902, -25.325) -> (0.7431, -25.4539) centre (0.7387, -25.304) ccw
  arc A368 (1.2563, -25.4338) -> (1.3986, -25.2932) centre (1.2489, -25.284) ccw
  arc A369 (1.4662, -24.9886) -> (1.3986, -25.2932) centre (2.3967, -25.3549) ccw
  arc A370 (1.9391, -24.6386) -> (1.4662, -24.9886) centre (1.9826, -25.1919) ccw
  line L62 (1.9979, -25.3863) -> (1.9391, -24.6386) construction
  arc A371 (2.5753, -25.2006) -> (2.4609, -24.9103) centre (1.5992, -25.4177) ccw
  arc A372 (2.4609, -24.9103) -> (1.9391, -24.6386) centre (1.9826, -25.1919) ccw
  arc A373 (2.5753, -25.2006) -> (2.7379, -25.3172) centre (2.7218, -25.168) ccw
  arc A374 (3.2479, -25.2568) -> (3.3788, -25.1055) centre (3.2288, -25.108) ccw
  arc A375 (3.4223, -24.7965) -> (3.3788, -25.1055) centre (4.3786, -25.0887) ccw
  arc A376 (3.8662, -24.4105) -> (3.4223, -24.7965) centre (3.9531, -24.9587) ccw
  line L63 (3.9836, -25.1513) -> (3.8662, -24.4105) construction
  arc A377 (4.5446, -24.9209) -> (4.4078, -24.6404) centre (3.5885, -25.2139) ccw
  arc A378 (4.4078, -24.6404) -> (3.8662, -24.4105) centre (3.9531, -24.9587) ccw
  arc A379 (4.5446, -24.9209) -> (4.7158, -25.0243) centre (4.688, -24.8769) ccw
  arc A380 (5.2196, -24.9241) -> (5.3381, -24.763) centre (5.1888, -24.7773) ccw
  arc A381 (5.3572, -24.4516) -> (5.3381, -24.763) centre (6.3336, -24.6678) ccw
  arc A382 (5.7696, -24.0319) -> (5.3572, -24.4516) centre (5.8991, -24.5716) ccw
  line L64 (5.9446, -24.7612) -> (5.7696, -24.0319) construction
  arc A383 (6.4859, -24.4875) -> (6.3274, -24.2186) centre (5.5557, -24.8546) ccw
  arc A384 (6.3274, -24.2186) -> (5.7696, -24.0319) centre (5.8991, -24.5716) ccw
  arc A385 (6.4859, -24.4875) -> (6.6647, -24.5772) centre (6.6254, -24.4324) ccw
  arc A386 (7.159, -24.4378) -> (7.2646, -24.2679) centre (7.1168, -24.2938) ccw
  arc A387 (7.2592, -23.9559) -> (7.2646, -24.2679) centre (8.2495, -24.0948) ccw
  arc A388 (7.6373, -23.5052) -> (7.2592, -23.9559) centre (7.8088, -24.033) ccw
  line L65 (7.8691, -24.2185) -> (7.6373, -23.5052) construction
  arc A389 (8.3871, -23.9031) -> (8.2081, -23.6475) centre (7.4886, -24.3421) ccw
  arc A390 (8.2081, -23.6475) -> (7.6373, -23.5052) centre (7.8088, -24.033) ccw
  arc A391 (8.3871, -23.9031) -> (8.5724, -23.9785) centre (8.5219, -23.8373) ccw
  arc A392 (9.0543, -23.8007) -> (9.1462, -23.6231) centre (9.001, -23.6605) ccw
  arc A393 (9.1164, -23.3125) -> (9.1462, -23.6231) centre (10.1145, -23.3733) ccw
  arc A394 (9.4579, -22.8335) -> (9.1164, -23.3125) centre (9.6703, -23.3462) ccw
  line L66 (9.745, -23.5264) -> (9.4579, -22.8335) construction
  arc A395 (10.2367, -23.1714) -> (10.0382, -22.9306) centre (9.3754, -23.6795) ccw
  arc A396 (10.0382, -22.9306) -> (9.4579, -22.8335) centre (9.6703, -23.3462) ccw
  arc A397 (10.2367, -23.1714) -> (10.4273, -23.232) centre (10.3659, -23.0952) ccw
  arc A398 (10.8938, -23.017) -> (10.9714, -22.8327) centre (10.8296, -22.8814) ccw
  arc A399 (10.9173, -22.5253) -> (10.9714, -22.8327) centre (11.9172, -22.5077) ccw
  arc A400 (11.2203, -22.021) -> (10.9173, -22.5253) centre (11.4722, -22.5155) ccw
  line L67 (11.5608, -22.6893) -> (11.2203, -22.021) construction
  arc A401 (12.0232, -22.2968) -> (11.8063, -22.0724) centre (11.2044, -22.8709) ccw
  arc A402 (11.8063, -22.0724) -> (11.2203, -22.021) centre (11.4722, -22.5155) ccw
  arc A403 (12.0232, -22.2968) -> (12.2179, -22.3423) centre (12.146, -22.2107) ccw
  arc A404 (12.6661, -22.0913) -> (12.7291, -21.9015) centre (12.5915, -21.9612) ccw
  arc A405 (12.651, -21.5993) -> (12.7291, -21.9015) centre (13.6464, -21.5033) ccw
  arc A406 (12.9134, -21.0728) -> (12.651, -21.5993) centre (13.2034, -21.546) ccw
  line L68 (13.3053, -21.7123) -> (12.9134, -21.0728) construction
  arc A407 (13.7355, -21.2847) -> (13.5017, -21.078) centre (12.9643, -21.9213) ccw
  arc A408 (13.5017, -21.078) -> (12.9134, -21.0728) centre (13.2034, -21.546) ccw
  arc A409 (13.7355, -21.2847) -> (13.9332, -21.3148) centre (13.8512, -21.1892) ccw
  arc A410 (14.3603, -21.0294) -> (14.4082, -20.8352) centre (14.2757, -20.9056) ccw
  arc A411 (14.3067, -20.5402) -> (14.4082, -20.8352) centre (15.2914, -20.3663) ccw
  arc A412 (14.527, -19.9947) -> (14.3067, -20.5402) centre (14.8532, -20.4437) ccw
  line L69 (14.9678, -20.6014) -> (14.527, -19.9947) construction
  arc A413 (15.3631, -20.1414) -> (15.1139, -19.9537) centre (14.6442, -20.8366) ccw
  arc A414 (15.1139, -19.9537) -> (14.527, -19.9947) centre (14.8532, -20.4437) ccw
  arc A415 (15.3631, -20.1414) -> (15.5626, -20.1559) centre (15.4709, -20.0372) ccw
  arc A416 (15.966, -19.8379) -> (15.9985, -19.6406) centre (15.8719, -19.7211) ccw
  arc A417 (15.8741, -19.3544) -> (15.9985, -19.6406) centre (16.8422, -19.1038) ccw
  arc A418 (16.051, -18.7933) -> (15.8741, -19.3544) centre (16.4114, -19.2153) ccw
  line L70 (16.5381, -19.3636) -> (16.051, -18.7933) construction
  arc A419 (16.896, -18.874) -> (16.6328, -18.7064) centre (16.2339, -19.6234) ccw
  arc A420 (16.6328, -18.7064) -> (16.051, -18.7933) centre (16.4114, -19.2153) ccw
  arc A421 (16.896, -18.874) -> (17.0961, -18.8727) centre (16.9954, -18.7616) ccw
  arc A422 (17.4732, -18.5241) -> (17.4901, -18.3248) centre (17.3703, -18.415) ccw
  arc A423 (17.3437, -18.0492) -> (17.4901, -18.3248) centre (18.2892, -17.7235) ccw
  arc A424 (17.476, -17.476) -> (17.3437, -18.0492) centre (17.8684, -17.8684) ccw
  line L71 (18.0063, -18.0063) -> (17.476, -17.476) construction
  arc A425 (18.3248, -17.4901) -> (18.0492, -17.3437) centre (17.7235, -18.2892) ccw
  arc A426 (18.0492, -17.3437) -> (17.476, -17.476) centre (17.8684, -17.8684) ccw
  arc A427 (18.3248, -17.4901) -> (18.5241, -17.4732) centre (18.415, -17.3703) ccw
  arc A428 (18.8727, -17.0961) -> (18.874, -16.896) centre (18.7616, -16.9954) ccw
  arc A429 (18.7064, -16.6328) -> (18.874, -16.896) centre (19.6234, -16.2339) ccw
  arc A430 (18.7933, -16.051) -> (18.7064, -16.6328) centre (19.2153, -16.4114) ccw
  line L72 (19.3636, -16.5381) -> (18.7933, -16.051) construction
  arc A431 (19.6406, -15.9985) -> (19.3544, -15.8741) centre (19.1038, -16.8422) ccw
  arc A432 (19.3544, -15.8741) -> (18.7933, -16.051) centre (19.2153, -16.4114) ccw
  arc A433 (19.6406, -15.9985) -> (19.8379, -15.966) centre (19.7211, -15.8719) ccw
  arc A434 (20.1559, -15.5626) -> (20.1414, -15.3631) centre (20.0372, -15.4709) ccw
  arc A435 (19.9537, -15.1139) -> (20.1414, -15.3631) centre (20.8366, -14.6442) ccw
  arc A436 (19.9947, -14.527) -> (19.9537, -15.1139) centre (20.4437, -14.8532) ccw
  line L73 (20.6014, -14.9678) -> (19.9947, -14.527) construction
  arc A437 (20.8352, -14.4082) -> (20.5402, -14.3067) centre (20.3663, -15.2914) ccw
  arc A438 (20.5402, -14.3067) -> (19.9947, -14.527) centre (20.4437, -14.8532) ccw
  arc A439 (20.8352, -14.4082) -> (21.0294, -14.3603) centre (20.9056, -14.2757) ccw
  arc A440 (21.3148, -13.9332) -> (21.2847, -13.7355) centre (21.1892, -13.8512) ccw
  arc A441 (21.078, -13.5017) -> (21.2847, -13.7355) centre (21.9213, -12.9643) ccw
  arc A442 (21.0728, -12.9134) -> (21.078, -13.5017) centre (21.546, -13.2034) ccw
  line L74 (21.7123, -13.3053) -> (21.0728, -12.9134) construction
  arc A443 (21.9015, -12.7291) -> (21.5993, -12.651) centre (21.5033, -13.6464) ccw
  arc A444 (21.5993, -12.651) -> (21.0728, -12.9134) centre (21.546, -13.2034) ccw
  arc A445 (21.9015, -12.7291) -> (22.0913, -12.6661) centre (21.9612, -12.5915) ccw
  arc A446 (22.3423, -12.2179) -> (22.2968, -12.0232) centre (22.2107, -12.146) ccw
  arc A447 (22.0724, -11.8063) -> (22.2968, -12.0232) centre (22.8709, -11.2044) ccw
  arc A448 (22.021, -11.2203) -> (22.0724, -11.8063) centre (22.5155, -11.4722) ccw
  line L75 (22.6893, -11.5608) -> (22.021, -11.2203) construction
  arc A449 (22.8327, -10.9714) -> (22.5253, -10.9173) centre (22.5077, -11.9172) ccw
  arc A450 (22.5253, -10.9173) -> (22.021, -11.2203) centre (22.5155, -11.4722) ccw
  arc A451 (22.8327, -10.9714) -> (23.017, -10.8938) centre (22.8814, -10.8296) ccw
  arc A452 (23.232, -10.4273) -> (23.1714, -10.2367) centre (23.0952, -10.3659) ccw
  arc A453 (22.9306, -10.0382) -> (23.1714, -10.2367) centre (23.6795, -9.3754) ccw
  arc A454 (22.8335, -9.4579) -> (22.9306, -10.0382) centre (23.3462, -9.6703) ccw
  line L76 (23.5264, -9.745) -> (22.8335, -9.4579) construction
  arc A455 (23.6231, -9.1462) -> (23.3125, -9.1164) centre (23.3733, -10.1145) ccw
  arc A456 (23.3125, -9.1164) -> (22.8335, -9.4579) centre (23.3462, -9.6703) ccw
  arc A457 (23.6231, -9.1462) -> (23.8007, -9.0543) centre (23.6605, -9.001) ccw
  arc A458 (23.9785, -8.5724) -> (23.9031, -8.3871) centre (23.8373, -8.5219) ccw
  arc A459 (23.6475, -8.2081) -> (23.9031, -8.3871) centre (24.3421, -7.4886) ccw
  arc A460 (23.5052, -7.6373) -> (23.6475, -8.2081) centre (24.033, -7.8088) ccw
  line L77 (24.2185, -7.8691) -> (23.5052, -7.6373) construction
  arc A461 (24.2679, -7.2646) -> (23.9559, -7.2592) centre (24.0948, -8.2495) ccw
  arc A462 (23.9559, -7.2592) -> (23.5052, -7.6373) centre (24.033, -7.8088) ccw
  arc A463 (24.2679, -7.2646) -> (24.4378, -7.159) centre (24.2938, -7.1168) ccw
  arc A464 (24.5772, -6.6647) -> (24.4875, -6.4859) centre (24.4324, -6.6254) ccw
  arc A465 (24.2186, -6.3274) -> (24.4875, -6.4859) centre (24.8546, -5.5557) ccw
  arc A466 (24.0319, -5.7696) -> (24.2186, -6.3274) centre (24.5716, -5.8991) ccw
  line L78 (24.7612, -5.9446) -> (24.0319, -5.7696) construction
  arc A467 (24.763, -5.3381) -> (24.4516, -5.3572) centre (24.6678, -6.3336) ccw
  arc A468 (24.4516, -5.3572) -> (24.0319, -5.7696) centre (24.5716, -5.8991) ccw
  arc A469 (24.763, -5.3381) -> (24.9241, -5.2196) centre (24.7773, -5.1888) ccw
  arc A470 (25.0243, -4.7158) -> (24.9209, -4.5446) centre (24.8769, -4.688) ccw
  arc A471 (24.6404, -4.4078) -> (24.9209, -4.5446) centre (25.2139, -3.5885) ccw
  arc A472 (24.4105, -3.8662) -> (24.6404, -4.4078) centre (24.9587, -3.9531) ccw
  line L79 (25.1513, -3.9836) -> (24.4105, -3.8662) construction
  arc A473 (25.1055, -3.3788) -> (24.7965, -3.4223) centre (25.0887, -4.3786) ccw
  arc A474 (24.7965, -3.4223) -> (24.4105, -3.8662) centre (24.9587, -3.9531) ccw
  arc A475 (25.1055, -3.3788) -> (25.2568, -3.2479) centre (25.108, -3.2288) ccw
  arc A476 (25.3172, -2.7379) -> (25.2006, -2.5753) centre (25.168, -2.7218) ccw
  arc A477 (24.9103, -2.4609) -> (25.2006, -2.5753) centre (25.4177, -1.5992) ccw
  arc A478 (24.6386, -1.9391) -> (24.9103, -2.4609) centre (25.1919, -1.9826) ccw
  line L80 (25.3863, -1.9979) -> (24.6386, -1.9391) construction
  arc A479 (25.2932, -1.3986) -> (24.9886, -1.4662) centre (25.3549, -2.3967) ccw
  arc A480 (24.9886, -1.4662) -> (24.6386, -1.9391) centre (25.1919, -1.9826) ccw
  arc A481 (25.2932, -1.3986) -> (25.4338, -1.2563) centre (25.284, -1.2489) ccw
  point P0 (25.4539, -0.7431)
  point P1 (-25.3172, 2.7379)
  point P2 (-24.9241, 5.2196)
  point P3 (-24.4378, 7.159)
  point P4 (-23.9785, 8.5724)
  point P5 (-23.8007, 9.0543)
  point P6 (-23.232, 10.4273)
  point P7 (-23.017, 10.8938)
  point P8 (-22.3423, 12.2179)
  point P9 (-22.0913, 12.6661)
  point P10 (-19.8379, 15.966)
  point P11 (-18.5241, 17.4732)
  point P12 (-17.4732, 18.5241)
  point P13 (-17.0961, 18.8727)
  point P14 (-15.966, 19.8379)
  point P15 (-15.5626, 20.1559)
  point P16 (-14.3603, 21.0294)
  point P17 (-13.9332, 21.3148)
  point P18 (-12.6661, 22.0913)
  point P19 (-10.4273, 23.232)
  point P20 (-9.0543, 23.8007)
  point P21 (-8.5724, 23.9785)
  point P22 (-7.159, 24.4378)
  point P23 (-6.6647, 24.5772)
  point P24 (-5.2196, 24.9241)
  point P25 (-4.7158, 25.0243)
  point P26 (-3.2479, 25.2568)
  point P27 (-2.7379, 25.3172)
  point P28 (-0.7431, 25.4539)
  point P29 (0.7431, 25.4539)
  point P30 (2.7379, 25.3172)
  point P31 (3.2479, 25.2568)
  point P32 (4.7158, 25.0243)
  point P33 (5.2196, 24.9241)
  point P34 (7.159, 24.4378)
  point P35 (9.0543, 23.8007)
  point P36 (10.4273, 23.232)
  point P37 (10.8938, 23.017)
  point P38 (12.2179, 22.3423)
  point P39 (12.6661, 22.0913)
  point P40 (15.966, 19.8379)
  point P41 (18.5241, 17.4732)
  point P42 (18.8727, 17.0961)
  point P43 (19.8379, 15.966)
  point P44 (20.1559, 15.5626)
  point P45 (21.0294, 14.3603)
  point P46 (21.3148, 13.9332)
  point P47 (22.0913, 12.6661)
  point P48 (23.232, 10.4273)
  point P49 (23.8007, 9.0543)
  point P50 (23.9785, 8.5724)
  point P51 (24.4378, 7.159)
  point P52 (24.5772, 6.6647)
  point P53 (25.0243, 4.7158)
  point P54 (25.2568, 3.2479)
  point P55 (25.3172, 2.7379)
  point P56 (25.4338, 1.2563)
  point P57 (2.7379, -25.3172)
  point P58 (3.2479, -25.2568)
  point P59 (4.7158, -25.0243)
  point P60 (5.2196, -24.9241)
  point P61 (6.6647, -24.5772)
  point P62 (9.0543, -23.8007)
  point P63 (10.4273, -23.232)
  point P64 (13.9332, -21.3148)
  point P65 (14.3603, -21.0294)
  point P66 (15.5626, -20.1559)
  point P67 (15.966, -19.8379)
  point P68 (17.4732, -18.5241)
  point P69 (18.5241, -17.4732)
  point P70 (18.8727, -17.0961)
  point P71 (19.8379, -15.966)
  point P72 (20.1559, -15.5626)
  point P73 (21.3148, -13.9332)
  point P74 (22.0913, -12.6661)
  point P75 (22.3423, -12.2179)
  point P76 (23.017, -10.8938)
  point P77 (23.8007, -9.0543)
  point P78 (24.4378, -7.159)
  point P79 (24.9241, -5.2196)
  point P80 (25.3172, -2.7379)
  point P81 (7.159, -24.4378)
  point P82 (-14.3603, -21.0294)
  point P83 (-22.3423, -12.2179)
  point P84 (-13.9332, -21.3148)
  point P85 (-12.6661, -22.0913)
  point P86 (-19.8379, -15.966)
  point P87 (-18.8727, -17.0961)
  point P88 (-2.7379, -25.3172)
  point P89 (-5.2196, -24.9241)
  point P90 (-7.159, -24.4378)
  point P91 (-9.0543, -23.8007)
  point P92 (-12.2179, -22.3423)
  point P93 (-10.8938, -23.017)
  point P94 (-18.5241, -17.4732)
  point P95 (-17.4732, -18.5241)
  point P96 (-21.0294, -14.3603)
  point P97 (-20.1559, -15.5626)
  point P98 (-21.3148, -13.9332)
  point P99 (-23.8007, -9.0543)
  point P100 (-24.4378, -7.159)
  point P101 (-24.5772, -6.6647)
  point P102 (-25.2568, -3.2479)
  point P103 (-25.0243, -4.7158)
  point P104 (-25.3172, -2.7379)
  dimension "d9" = 0.15
  dimension "d10" = 1
  dimension "d11" = 0.555
  dimension "d12" = 0.75
  dimension "d13" = 0.4
  dimension "d18" = 0.9
  dimension "d21" = 360
  constraints: 960 point on circle, 481 centre point, 162 end point, 5 symmetric about line, 2 coincident, 2 horizontal, 2 tangent, 1 line through centre, 1608 other
  measures "d9" radius of A4
  measures "d10" radius of A3
  measures "d11" radius of A2
  measures "d12" distance of L0.start L0.end
  measures "d13" distance from line of A3.centre L0